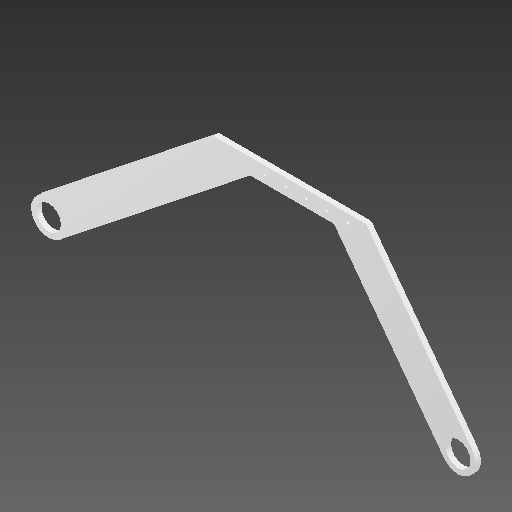
# Autodesk Inventor part: motor_support_mount
Saved by Autodesk Inventor 2020.2 (Build 242310000, 310)
## iProperties
Created: 2020-03-28
Part Number: motor_support_mount
Material: Aluminum 6061
Document SubType Name: Modeling
Designer: agmle
Density: 2.7 g/cm^3
Appearance: Aluminum - Flat
Mass: 406.082 g
Surface Area: 578.279 cm^2
Volume: 150.401 cm^3
Author: agmle
Autodesk Inventor part; units mm, degrees
ref_plane "YZ Plane" through (0, 0, 0) normal (1, 0, 0) x (0, 1, 0)
ref_plane "XZ Plane" through (0, 0, 0) normal (0, 1, 0) x (-1, 0, 0)
ref_plane "XY Plane" through (0, 0, 0) normal (0, 0, 1) x (1, 0, 0)
sketch "Sketch1" plane through (0, 0, 0) normal (0, 0, 1) x (1, 0, 0)
  line L0 (-245.3259, 0) -> (63.2798, 244.4632) construction
  line L1 (63.2798, 244.4632) -> (245.3259, 0) construction
  line L2 (245.3259, 0) -> (-245.3259, 0) construction
  circle A0 centre (-245.3259, 0) radius 14.7955 construction
  circle A1 centre (245.3259, 0) radius 14.7955 construction
  arc A2 (-258.4559, 16.5751) -> (-232.1959, -16.5751) centre (-245.3259, 0) ccw
  arc A3 (228.3663, -12.6295) -> (262.2855, 12.6295) centre (245.3259, 0) ccw
  line L3 (-258.4559, 16.5751) -> (-47.8104, 183.4388)
  line L4 (-47.8104, 183.4388) -> (135.0877, 183.4388)
  line L5 (135.0877, 183.4388) -> (262.2855, 12.6295)
  line L6 (228.3663, -12.6295) -> (96.5448, 164.3888)
  line L7 (96.5448, 164.3888) -> (-3.7505, 164.3888)
  line L8 (-3.7505, 164.3888) -> (-232.1959, -16.5751)
  point P0 (0, 0)
  point P1 (0, 0)
  dimension "d0" = 304.8
  dimension "d1" = 393.7
  dimension "d2" = 490.6518
  dimension "d3" = 29.591
  dimension "d4" = 6.35
  dimension "d5" = 19.05
  dimension "d6" = 164.3888
  constraints: 18 end point, 5 coincident, 5 parallel, 4 centre point, 4 point on circle, 4 tangent, 2 equal radius, 2 horizontal, 1 midpoint
  measures "d0" distance of L0.end L1.end
  measures "d1" distance of L0.start L0.end
  measures "d2" distance of L1.end L0.start
  measures "d3" diameter of A0
  measures "d4" radial gap between concentric circles of A0 A2
  measures "d5" distance between parallel lines of L7 L4
  measures "d6" distance between parallel lines of L2 L7
extrude "Frame" add sketch "Sketch1" along normal blind 6.35
sketch "Sketch2" plane through (0, 0, 6.35) normal (0, 0, 1) x (1, 0, 0)
  arc A0 (-258.4559, 16.5751) -> (-232.1959, -16.5751) centre (-245.3259, 0) ccw projected
  arc A1 (228.3663, -12.6295) -> (262.2855, 12.6295) centre (245.3259, 0) ccw projected
  point P0 (0, 0)
  point P1 (-245.3259, 0)
  point P2 (245.3259, 0)
  constraints: 2 coincident
hole "Struts" at (-245.3259, 0, 6.35) at (245.3259, 0, 6.35) direction (0, 0, -1) diameter 29.591 end through all start extended yes
fillet "Edge Break" radius 5 4 edges at (96.5448, 164.3888, 3.175) (-3.7505, 164.3888, 3.175) (-47.8104, 183.4388, 3.175) (135.0877, 183.4388, 3.175)
sketch "Sketch3" plane through (0, 0, 0) normal (0, 0, -1) x (-1, 0, 0)
  line L0 (2.01, 164.3888) -> (-94.0341, 164.3888) construction
  line L1 (-1.2532, 164.3888) -> (-125.3068, 164.3888) construction
  line L2 (-125.3068, 164.3888) -> (-125.3068, 189.7888) construction
  line L3 (-125.3068, 189.7888) -> (-1.2532, 189.7888) construction
  line L4 (-1.2532, 189.7888) -> (-1.2532, 164.3888) construction
  arc A0 (5.1147, 163.3081) -> (2.01, 164.3888) centre (2.01, 159.3888) ccw construction
  line L5 (-112.81, 173.9138) -> (-88.045, 173.9138) construction
  line L6 (-88.045, 173.9138) -> (-63.28, 173.9138) construction
  line L7 (-63.28, 173.9138) -> (-38.515, 173.9138) construction
  line L8 (-38.515, 173.9138) -> (-13.75, 173.9138) construction
  line L9 (-63.28, 164.3888) -> (-63.28, 173.9138) construction
  point P0 (0, 0)
  dimension "d17" = 25.4
  dimension "d18" = 3.2632
  dimension "d19" = 124.0536
  dimension "d21" = 9.525
  dimension "d31" = 24.765
  constraints: 18 end point, 5 equal length, 3 collinear, 2 horizontal, 2 perpendicular, 1 midpoint, 1 point on line
  measures "d17" distance of L1.end L2.end
  measures "d18" distance from line of A0.centre L4
  measures "d19" distance of L2.end L3.end
  measures "d21" distance from line of L1 L6.end
  measures "d31" distance of L5.start L5.end
hole "Mount Bolts" at (112.81, 173.9138, 0) at (88.045, 173.9138, 0) at (63.28, 173.9138, 0) at (38.515, 173.9138, 0) at (13.75, 173.9138, 0) direction (0, 0, 1) diameter 3.4036 end through all start extended yes countersink diameter 6.2992 countersink angle 90 clearance for "Flat Head Machine Screw" size "M3" standard "Ansi Metric M Profile"
body "Solid1"
